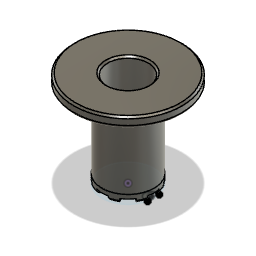
transfer rod handle v4 (Autodesk Fusion 360 design; units mm, degrees)
Autodesk Fusion 360 part; units mm, degrees
note: some values were not read from the file. Set by a fixed rule: which sketch regions a step uses.
sketch "Sketch1" plane through (0, 0, 0) normal (0, 0, 1) x (1, 0, 0)
  line L0 (93.1435, 165) -> (35, 165)
  line L1 (35, 165) -> (35, 15)
  line L2 (35, 15) -> (45, 15)
  line L3 (45, 15) -> (45, 150)
  line L4 (93.1435, 145) -> (93.1435, 165)
  line L5 (45, 15) -> (45, 0)
  line L6 (45, 0) -> (0, 0)
  line L7 (0, 0) -> (0, 15)
  line L8 (0, 15) -> (35, 15)
  line L9 (45, 150) -> (78.1435, 150)
  line L10 (78.1435, 150) -> (93.1435, 145)
  dimension "d1" = 35
  dimension "d2" = 150
  dimension "d3" = 10
  dimension "d5" = 20
  dimension "d6" = 15
  dimension "d24" = 15
  dimension "d25" = 15
  constraint perpendicular L0 L1
  constraint perpendicular L1 L2
  constraint perpendicular L2 L3
  constraint perpendicular L2 L5
  constraint perpendicular L3 L6
  constraint perpendicular L2 L7
  constraint perpendicular L1 L8
  constraint coincident L6.end L7.start
  constraint horizontal L6
  constraint perpendicular L3 L9
  constraint vertical L4
  measures "d1" distance of L6.end L1
  measures "d2" distance of L0.end L1.end
  measures "d3" distance of L1 L3
  measures "d5" distance of L0.start L4.start
  measures "d6" distance of L2.end L5.end
  measures "d24" distance of L0 L9
  measures "d25" distance of L4 L9.end
revolve "Revolve1" add sketch "Sketch1" angle 360 about axis through (0, 1.75, 0) along (0, 1, 0) contours L0 L1 L2 L3 L4 L9 L10 makes body 1
revolve "Revolve2" add sketch "Sketch1" angle 360 about axis through (0, 0, 0) along (0, 1, 0) separate body contours L2 L5 L6 L7 L8 makes body 2
fillet "Fillet2" radius 10 1 edges at (-41.9547, 150, -16.2727) on bodies 1
sketch "Sketch2" plane through (0, 0, 0) normal (0, -1, 0) x (1, 0, 0)
  circle A0 centre (0, 0) radius 45
  line L0 (43.8748, 10) -> (39, 10)
  line L1 (39, -10) -> (43.8748, -10)
  arc A1 (39, 10) -> (39, -10) centre (39, 0) ccw
  dimension "d30" = 39
  dimension "d37" = 10
  constraint coincident A0 L0.start
  constraint horizontal L0
  constraint coincident A0 L1.end
  constraint parallel L0 L1
  constraint tangent L0 A1
  constraint tangent L1 A1
  constraint horizontal A0.centre A1.centre
  measures "d30" distance of A0.centre A1.centre
  measures "d37" radius of A1
chamfer "Chamfer2" distance 5 angle 45 1 edges at (-41.9547, 0, -16.2727) on bodies 2
extrude "Extrude4" cut sketch "Sketch2" against normal blind 8 contours A0 L0 L1 A1 picked at (40.3521, -3.1977) bodies 2
hole "Hole2" at (39, 0, 0) direction (0, 1, 0) diameter 4.234 depth 50 tip angle 118 bodies 1 2
thread "Thread2" "ISO Metric profile 5.0 M5x0.8 6H" thread offset 0 thread depth 10
pattern_circular "C-Pattern2" count 8 over 360 about axis through (0, 1.75, 0) along (0, 1, 0) of "Extrude4", "Hole2"
fillet "Fillet3" radius 5 1 edges at (-86.8402, 145, -33.6821) on bodies 1
chamfer "Chamfer3" distance 3 angle 45 2 edges at (-86.8402, 165, -33.6821) (-32.6315, 165, -12.6565) on bodies 1
hole "Hole3" at (0, 0, 0) direction (0, 1, 0) diameter 45 end through all bodies 1 2
